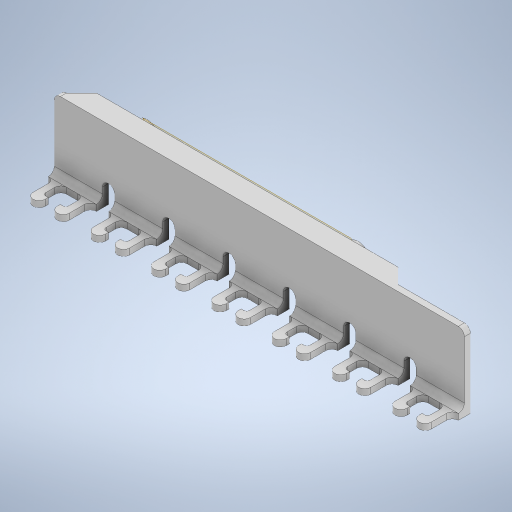
# Autodesk Inventor part: DCB2_CableClip
Saved by Autodesk Inventor 2024.3 (Build 283343000, 343)
## iProperties
Created: 2024-05-18
Part Number: DCB2_CableClip
Material: Generic
Document SubType Name: Modeling
Designer: atrus
Density: 1 g/cm^3
Appearance: Default
Author: atrus
Autodesk Inventor part; units mm, degrees
ref_plane "YZ Plane" through (0, 0, 0) normal (1, 0, 0) x (0, 1, 0)
ref_plane "XZ Plane" through (0, 0, 0) normal (0, 1, 0) x (-1, 0, 0)
ref_plane "XY Plane" through (0, 0, 0) normal (0, 0, 1) x (1, 0, 0)
ref_plane "Work Plane1" through (0, 0, 0) normal (0, 0, 1) x (1, 0, 0)
sketch "Sketch1" plane through (0, 0, 0) normal (0, 0, 1) x (1, 0, 0)
  line L0 (19.6661, -71) -> (82.3339, -71) construction
  line L1 (82.3339, -81) -> (19.6661, -81) construction
  line L2 (1, -71) -> (101, -71)
  line L3 (101, -71) -> (101, -81)
  line L4 (101, -81) -> (1, -81)
  line L5 (1, -81) -> (1, -71)
  point P0 (0, 0)
  point P1 (51, -71)
  point P2 (51, -81)
  point P3 (101, -76)
  point P4 (1, -76)
  dimension "d0" = 100
  constraints: 8 end point, 6 midpoint, 2 parallel, 1 horizontal, 1 perpendicular
  measures "d0" distance of point (101, -76) point (1, -76)
extrude "Extrusion1" add sketch "Sketch1" along normal blind 5
sketch "Sketch2" plane through (0, 0, 5) normal (0, 0, 1) x (1, 0, 0)
  line L0 (130.0002, -96) -> (-5.9998, -96)
  line L1 (-5.9998, -96) -> (-5.9998, -71)
  line L2 (-5.9998, -71) -> (130.0002, -71)
  line L3 (130.0002, -71) -> (130.0002, -96)
  line L4 (-2.4998, -51.4004) -> (-2.4998, -61.4004) projected
  line L5 (126.5002, -51.4004) -> (126.5002, -61.4004) projected
  line L6 (101, -71) -> (1, -71) projected
  point P0 (0, 0)
  point P1 (-2.4998, -56.4004)
  point P2 (130.0002, -83.5)
  point P3 (51, -71)
  dimension "d3" = 3.5
  dimension "d4" = 3.5
  dimension "d5" = 25
  constraints: 8 end point, 3 midpoint, 2 parallel, 1 horizontal, 1 perpendicular, 1 point on line
  measures "d3" distance from line of point (-2.5, -56.4) L1
  measures "d4" distance from line of point (130, -83.5) L5
  measures "d5" distance of L0.end L1.end
extrude "Extrusion2" add sketch "Sketch2" along normal blind 2
sketch "Sketch3" plane through (0, 0, 7) normal (0, 0, 1) x (1, 0, 0)
  line L0 (-2.4998, -63.9004) -> (6.5002, -63.9004)
  line L1 (17.5002, -63.9004) -> (26.5002, -63.9004)
  line L2 (37.5002, -63.9004) -> (46.5002, -63.9004)
  line L3 (57.5002, -63.9004) -> (66.5002, -63.9004)
  line L4 (77.5002, -63.9004) -> (86.5002, -63.9004)
  line L5 (97.5002, -63.9004) -> (106.5002, -63.9004)
  line L6 (117.5002, -63.9004) -> (126.5002, -63.9004)
  line L7 (2.0002, -63.9004) -> (2.0002, -96) construction
  line L8 (-5.9998, -96) -> (130.0002, -96) construction
  line L9 (22.0002, -63.9004) -> (22.0002, -96) construction
  line L10 (42.0002, -63.9004) -> (42.0002, -111) construction
  line L11 (62.0002, -63.9004) -> (62.0002, -96) construction
  line L12 (82.0002, -63.9004) -> (82.0002, -96) construction
  line L13 (102.0002, -63.9004) -> (102.0002, -96) construction
  line L14 (122.0002, -63.9004) -> (122.0002, -96) construction
  line L15 (-5.9998, -94) -> (10.0002, -94)
  line L16 (10.0002, -94) -> (10.0002, -96)
  line L17 (10.0002, -96) -> (-5.9998, -96)
  line L18 (-5.9998, -96) -> (-5.9998, -94)
  line L19 (30.0002, -94) -> (30.0002, -96)
  line L20 (14.0002, -94) -> (30.0002, -94)
  line L21 (30.0002, -96) -> (14.0002, -96)
  line L22 (14.0002, -96) -> (14.0002, -94)
  line L23 (50.0002, -94) -> (50.0002, -96)
  line L24 (34.0002, -94) -> (50.0002, -94)
  line L25 (50.0002, -96) -> (34.0002, -96)
  line L26 (34.0002, -96) -> (34.0002, -94)
  line L27 (70.0002, -94) -> (70.0002, -96)
  line L28 (54.0002, -94) -> (70.0002, -94)
  line L29 (70.0002, -96) -> (54.0002, -96)
  line L30 (54.0002, -96) -> (54.0002, -94)
  line L31 (90.0002, -94) -> (90.0002, -96)
  line L32 (74.0002, -94) -> (90.0002, -94)
  line L33 (90.0002, -96) -> (74.0002, -96)
  line L34 (74.0002, -96) -> (74.0002, -94)
  line L35 (110.0002, -94) -> (110.0002, -96)
  line L36 (94.0002, -94) -> (110.0002, -94)
  line L37 (110.0002, -96) -> (94.0002, -96)
  line L38 (94.0002, -96) -> (94.0002, -94)
  line L39 (130.0002, -94) -> (130.0002, -96)
  line L40 (114.0002, -94) -> (130.0002, -94)
  line L41 (130.0002, -96) -> (114.0002, -96)
  line L42 (114.0002, -96) -> (114.0002, -94)
  point P0 (0, 0)
  point P1 (2.0002, -94)
  point P2 (22.0002, -94)
  point P3 (22.0002, -96)
  point P4 (42.0002, -94)
  point P5 (42.0002, -96)
  point P6 (62.0002, -94)
  point P7 (62.0002, -96)
  point P8 (82.0002, -94)
  point P9 (82.0002, -96)
  point P10 (102.0002, -94)
  point P11 (122.0002, -94)
  point P12 (122.0002, -96)
extrude "Extrusion3" add sketch "Sketch3" along normal blind 2
sketch "Sketch4" plane through (-5.9998, -96, 5) normal (0, -1, 0) x (1, 0, 0)
  line L0 (0, 4) -> (16, 4) construction
  line L1 (8, 4) -> (8, 21.3357) construction
  line L2 (2, 4) -> (2, 11)
  line L3 (4, 13) -> (4, 13)
  line L4 (6, 11) -> (6, 10)
  line L5 (6, 10) -> (5.2, 10)
  line L6 (4.2, 9) -> (4.2, 6)
  arc A0 (5.2, 10) -> (4.2, 9) centre (5.2, 9) ccw
  arc A1 (6, 11) -> (4, 13) centre (4, 11) ccw
  arc A2 (4, 13) -> (2, 11) centre (4, 11) ccw
  line L7 (0, 2) -> (0, 4) projected
  line L8 (2, 4) -> (4.2, 4)
  arc A3 (4.2, 6) -> (6.2, 4) centre (6.2, 6) ccw
  line L9 (4.2, 4) -> (6.2, 4)
  line L10 (14, 4) -> (14, 11)
  line L11 (12, 13) -> (12, 13)
  line L12 (10, 11) -> (10, 10)
  line L13 (10, 10) -> (10.8, 10)
  line L14 (11.8, 9) -> (11.8, 6)
  arc A4 (11.8, 9) -> (10.8, 10) centre (10.8, 9) ccw
  arc A5 (12, 13) -> (10, 11) centre (12, 11) ccw
  arc A6 (14, 11) -> (12, 13) centre (12, 11) ccw
  line L15 (14, 4) -> (11.8, 4)
  arc A7 (9.8, 4) -> (11.8, 6) centre (9.8, 6) ccw
  line L16 (11.8, 4) -> (9.8, 4)
  line L17 (34, 4) -> (31.8, 4)
  arc A8 (26, 11) -> (24, 13) centre (24, 11) ccw
  line L18 (24, 13) -> (24, 13)
  arc A9 (24, 13) -> (22, 11) centre (24, 11) ccw
  line L19 (31.8, 4) -> (29.8, 4)
  arc A10 (29.8, 4) -> (31.8, 6) centre (29.8, 6) ccw
  line L20 (31.8, 9) -> (31.8, 6)
  arc A11 (31.8, 9) -> (30.8, 10) centre (30.8, 9) ccw
  line L21 (30, 10) -> (30.8, 10)
  line L22 (34, 4) -> (34, 11)
  line L23 (30, 11) -> (30, 10)
  line L24 (32, 13) -> (32, 13)
  arc A12 (34, 11) -> (32, 13) centre (32, 11) ccw
  arc A13 (32, 13) -> (30, 11) centre (32, 11) ccw
  line L25 (26, 11) -> (26, 10)
  line L26 (26, 10) -> (25.2, 10)
  arc A14 (25.2, 10) -> (24.2, 9) centre (25.2, 9) ccw
  line L27 (24.2, 9) -> (24.2, 6)
  line L28 (22, 4) -> (22, 11)
  line L29 (22, 4) -> (24.2, 4)
  line L30 (24.2, 4) -> (26.2, 4)
  arc A15 (24.2, 6) -> (26.2, 4) centre (26.2, 6) ccw
  line L31 (54, 4) -> (51.8, 4)
  arc A16 (46, 11) -> (44, 13) centre (44, 11) ccw
  line L32 (44, 13) -> (44, 13)
  arc A17 (44, 13) -> (42, 11) centre (44, 11) ccw
  line L33 (51.8, 4) -> (49.8, 4)
  arc A18 (49.8, 4) -> (51.8, 6) centre (49.8, 6) ccw
  line L34 (51.8, 9) -> (51.8, 6)
  arc A19 (51.8, 9) -> (50.8, 10) centre (50.8, 9) ccw
  line L35 (50, 10) -> (50.8, 10)
  line L36 (54, 4) -> (54, 11)
  line L37 (50, 11) -> (50, 10)
  line L38 (52, 13) -> (52, 13)
  arc A20 (54, 11) -> (52, 13) centre (52, 11) ccw
  arc A21 (52, 13) -> (50, 11) centre (52, 11) ccw
  line L39 (46, 11) -> (46, 10)
  line L40 (46, 10) -> (45.2, 10)
  arc A22 (45.2, 10) -> (44.2, 9) centre (45.2, 9) ccw
  line L41 (44.2, 9) -> (44.2, 6)
  line L42 (42, 4) -> (42, 11)
  line L43 (42, 4) -> (44.2, 4)
  line L44 (44.2, 4) -> (46.2, 4)
  arc A23 (44.2, 6) -> (46.2, 4) centre (46.2, 6) ccw
  line L45 (74, 4) -> (71.8, 4)
  arc A24 (66, 11) -> (64, 13) centre (64, 11) ccw
  line L46 (64, 13) -> (64, 13)
  arc A25 (64, 13) -> (62, 11) centre (64, 11) ccw
  line L47 (71.8, 4) -> (69.8, 4)
  arc A26 (69.8, 4) -> (71.8, 6) centre (69.8, 6) ccw
  line L48 (71.8, 9) -> (71.8, 6)
  arc A27 (71.8, 9) -> (70.8, 10) centre (70.8, 9) ccw
  line L49 (70, 10) -> (70.8, 10)
  line L50 (74, 4) -> (74, 11)
  line L51 (70, 11) -> (70, 10)
  line L52 (72, 13) -> (72, 13)
  arc A28 (74, 11) -> (72, 13) centre (72, 11) ccw
  arc A29 (72, 13) -> (70, 11) centre (72, 11) ccw
  line L53 (66, 11) -> (66, 10)
  line L54 (66, 10) -> (65.2, 10)
  arc A30 (65.2, 10) -> (64.2, 9) centre (65.2, 9) ccw
  line L55 (64.2, 9) -> (64.2, 6)
  line L56 (62, 4) -> (62, 11)
  line L57 (62, 4) -> (64.2, 4)
  line L58 (64.2, 4) -> (66.2, 4)
  arc A31 (64.2, 6) -> (66.2, 4) centre (66.2, 6) ccw
  line L59 (94, 4) -> (91.8, 4)
  arc A32 (86, 11) -> (84, 13) centre (84, 11) ccw
  line L60 (84, 13) -> (84, 13)
  arc A33 (84, 13) -> (82, 11) centre (84, 11) ccw
  line L61 (91.8, 4) -> (89.8, 4)
  arc A34 (89.8, 4) -> (91.8, 6) centre (89.8, 6) ccw
  line L62 (91.8, 9) -> (91.8, 6)
  arc A35 (91.8, 9) -> (90.8, 10) centre (90.8, 9) ccw
  line L63 (90, 10) -> (90.8, 10)
  line L64 (94, 4) -> (94, 11)
  line L65 (90, 11) -> (90, 10)
  line L66 (92, 13) -> (92, 13)
  arc A36 (94, 11) -> (92, 13) centre (92, 11) ccw
  arc A37 (92, 13) -> (90, 11) centre (92, 11) ccw
  line L67 (86, 11) -> (86, 10)
  line L68 (86, 10) -> (85.2, 10)
  arc A38 (85.2, 10) -> (84.2, 9) centre (85.2, 9) ccw
  line L69 (84.2, 9) -> (84.2, 6)
  line L70 (82, 4) -> (82, 11)
  line L71 (82, 4) -> (84.2, 4)
  line L72 (84.2, 4) -> (86.2, 4)
  arc A39 (84.2, 6) -> (86.2, 4) centre (86.2, 6) ccw
  line L73 (114, 4) -> (111.8, 4)
  arc A40 (106, 11) -> (104, 13) centre (104, 11) ccw
  line L74 (104, 13) -> (104, 13)
  arc A41 (104, 13) -> (102, 11) centre (104, 11) ccw
  line L75 (111.8, 4) -> (109.8, 4)
  arc A42 (109.8, 4) -> (111.8, 6) centre (109.8, 6) ccw
  line L76 (111.8, 9) -> (111.8, 6)
  arc A43 (111.8, 9) -> (110.8, 10) centre (110.8, 9) ccw
  line L77 (110, 10) -> (110.8, 10)
  line L78 (114, 4) -> (114, 11)
  line L79 (110, 11) -> (110, 10)
  line L80 (112, 13) -> (112, 13)
  arc A44 (114, 11) -> (112, 13) centre (112, 11) ccw
  arc A45 (112, 13) -> (110, 11) centre (112, 11) ccw
  line L81 (106, 11) -> (106, 10)
  line L82 (106, 10) -> (105.2, 10)
  arc A46 (105.2, 10) -> (104.2, 9) centre (105.2, 9) ccw
  line L83 (104.2, 9) -> (104.2, 6)
  line L84 (102, 4) -> (102, 11)
  line L85 (102, 4) -> (104.2, 4)
  line L86 (104.2, 4) -> (106.2, 4)
  arc A47 (104.2, 6) -> (106.2, 4) centre (106.2, 6) ccw
  line L87 (134, 4) -> (131.8, 4)
  arc A48 (126, 11) -> (124, 13) centre (124, 11) ccw
  line L88 (124, 13) -> (124, 13)
  arc A49 (124, 13) -> (122, 11) centre (124, 11) ccw
  line L89 (131.8, 4) -> (129.8, 4)
  arc A50 (129.8, 4) -> (131.8, 6) centre (129.8, 6) ccw
  line L90 (131.8, 9) -> (131.8, 6)
  arc A51 (131.8, 9) -> (130.8, 10) centre (130.8, 9) ccw
  line L91 (130, 10) -> (130.8, 10)
  line L92 (134, 4) -> (134, 11)
  line L93 (130, 11) -> (130, 10)
  line L94 (132, 13) -> (132, 13)
  arc A52 (134, 11) -> (132, 13) centre (132, 11) ccw
  arc A53 (132, 13) -> (130, 11) centre (132, 11) ccw
  line L95 (126, 11) -> (126, 10)
  line L96 (126, 10) -> (125.2, 10)
  arc A54 (125.2, 10) -> (124.2, 9) centre (125.2, 9) ccw
  line L97 (124.2, 9) -> (124.2, 6)
  line L98 (122, 4) -> (122, 11)
  line L99 (122, 4) -> (124.2, 4)
  line L100 (124.2, 4) -> (126.2, 4)
  arc A55 (124.2, 6) -> (126.2, 4) centre (126.2, 6) ccw
  point P0 (5.9998, -5)
  point P1 (4, 13)
  point P2 (5.6, 10)
  point P3 (12, 13)
  point P4 (10.4, 10)
  point P5 (24, 13)
  point P6 (28, 4)
  point P7 (30.4, 10)
  point P8 (32, 13)
  point P9 (25.6, 10)
  point P10 (44, 13)
  point P11 (48, 4)
  point P12 (50.4, 10)
  point P13 (52, 13)
  point P14 (45.6, 10)
  point P15 (64, 13)
  point P16 (68, 4)
  point P17 (70.4, 10)
  point P18 (72, 13)
  point P19 (65.6, 10)
  point P20 (84, 13)
  point P21 (88, 4)
  point P22 (90.4, 10)
  point P23 (92, 13)
  point P24 (85.6, 10)
  point P25 (104, 13)
  point P26 (108, 4)
  point P27 (110.4, 10)
  point P28 (112, 13)
  point P29 (105.6, 10)
  point P30 (124, 13)
  point P31 (128, 4)
  point P32 (130.4, 10)
  point P33 (132, 13)
  point P34 (125.6, 10)
  point P35 (4, 13)
  point P36 (132, 13)
  point P37 (124, 13)
  point P38 (112, 13)
  point P39 (104, 13)
  point P40 (92, 13)
  point P41 (84, 13)
  point P42 (72, 13)
  point P43 (64, 13)
  point P44 (52, 13)
  point P45 (44, 13)
  point P46 (32, 13)
  point P47 (24, 13)
  point P48 (12, 13)
  dimension "d19" = 1
  dimension "d20" = 2
  dimension "d21" = 4
  dimension "d22" = 9
  dimension "d23" = 6
  dimension "d24" = 2.2
  dimension "d70" = 2
  dimension "d71" = 2
  dimension "d74" = 20
  constraints: 198 end point, 112 point on circle, 56 centre point, 17 symmetric about line, 16 point on line, 8 tangent, 4 perpendicular, 3 midpoint, 2 collinear, 2 vertical, 1 concentric, 1 horizontal, 346 other
  measures "d19" radius of A0
  measures "d20" radius of A1
  measures "d21" distance from line of L2 L4.end
  measures "d22" distance from line of L0 point (4, 13)
  measures "d23" distance from line of L0 point (5.6, 10)
  measures "d24" distance between parallel lines of L2 L6
  measures "d70" distance from line of L0.start L2
  measures "d71" radius of A3
  measures "d74" distance of L16.start L17.end
extrude "Extrusion4" add sketch "Sketch4" against normal blind 2
fillet "Fillet1" radius 2 7 edges at (2.0002, -94, 7) (22.0002, -94, 7) (42.0002, -94, 7) (62.0002, -94, 7) (82.0002, -94, 7) (102.0002, -94, 7) (122.0002, -94, 7)
fillet "Fillet2" radius 2 2 edges at (-5.9998, -71, 6) (130.0002, -71, 6)
sketch "Sketch7" plane through (0, 0, 0) normal (0, 0, -1) x (-1, 0, 0)
  circle A0 centre (-16, -76) radius 4.2 construction
  circle A1 centre (-86, -76) radius 4.2 construction
  circle A2 centre (-16, -76) radius 4
  circle A3 centre (-86, -76) radius 4
  point P0 (0, 0)
  dimension "d52" = 0.2
  constraints: 2 centre point, 2 coincident, 1 equal radius
  measures "d52" radial gap between concentric circles of A0 A2
extrude "Extrusion6" add sketch "Sketch7" along normal blind 1.8
sketch "Sketch6" plane through (0, 0, -1.8) normal (0, 0, -1) x (-1, 0, 0)
  circle A0 centre (-16, -76) radius 1.8 construction
  line L0 (-1, -81) -> (-101, -81) construction
  line L1 (-1, -71) -> (-1, -81) construction
  line L2 (-101, -71) -> (-1, -71) construction
  line L3 (-101, -81) -> (-101, -71) construction
  circle A1 centre (-86, -76) radius 1.8 construction
  circle A2 centre (-16, -76) radius 2
  circle A3 centre (-86, -76) radius 2
  point P0 (0, 0)
  dimension "d51" = 4
  constraints: 2 centre point, 2 coincident, 1 equal radius
  measures "d51" diameter of A2
extrude "Extrusion7" cut sketch "Sketch6" against normal blind 7
sketch "Sketch9" plane through (0, 0, 5) normal (0, 0, -1) x (-1, 0, 0)
  line L0 (-130.0002, -96) -> (-130.0002, -73) construction
  line L1 (-130.0002, -88) -> (5.9998, -88) construction
  line L2 (5.9998, -73) -> (5.9998, -96) construction
  line L3 (-114.0002, -96) -> (-110.0002, -96)
  line L4 (-110.0002, -96) -> (-110.0002, -88)
  line L5 (-110.0002, -88) -> (-114.0002, -88)
  line L6 (-114.0002, -88) -> (-114.0002, -96)
  line L7 (-94.0002, -96) -> (-90.0002, -96)
  line L8 (-90.0002, -96) -> (-90.0002, -88)
  line L9 (-90.0002, -88) -> (-94.0002, -88)
  line L10 (-94.0002, -88) -> (-94.0002, -96)
  line L11 (-74.0002, -96) -> (-70.0002, -96)
  line L12 (-70.0002, -96) -> (-70.0002, -88)
  line L13 (-70.0002, -88) -> (-74.0002, -88)
  line L14 (-74.0002, -88) -> (-74.0002, -96)
  line L15 (-54.0002, -96) -> (-50.0002, -96)
  line L16 (-50.0002, -96) -> (-50.0002, -88)
  line L17 (-50.0002, -88) -> (-54.0002, -88)
  line L18 (-54.0002, -88) -> (-54.0002, -96)
  line L19 (-34.0002, -96) -> (-30.0002, -96)
  line L20 (-30.0002, -96) -> (-30.0002, -88)
  line L21 (-30.0002, -88) -> (-34.0002, -88)
  line L22 (-34.0002, -88) -> (-34.0002, -96)
  line L23 (-14.0002, -96) -> (-10.0002, -96)
  line L24 (-10.0002, -96) -> (-10.0002, -88)
  line L25 (-10.0002, -88) -> (-14.0002, -88)
  line L26 (-14.0002, -88) -> (-14.0002, -96)
  line L27 (5.9998, -96) -> (-130.0002, -96) projected
  point P0 (0, 0)
  dimension "d62" = 20
  dimension "d83" = 8
  constraints: 50 end point, 9 point on line, 3 horizontal, 2 parallel, 1 perpendicular, 46 other
  measures "d62" distance of L4.end L8.end
extrude "Extrusion9" cut sketch "Sketch9" against normal blind 2
fillet "Fillet4" radius 2 12 edges at (114.0002, -88, 6) (110.0002, -88, 6) (90.0002, -88, 6) (94.0002, -88, 6) (74.0002, -88, 6) (54.0002, -88, 6) (34.0002, -88, 6) (14.0002, -88, 6) (70.0002, -88, 6) (50.0002, -88, 6) (30.0002, -88, 6) (10.0002, -88, 6)
fillet "Fillet5" radius 2 14 edges at (-3.9998, -95, 9) (8.0002, -95, 9) (16.0002, -95, 9) (28.0002, -95, 9) (48.0002, -95, 9) (68.0002, -95, 9) (88.0002, -95, 9) (108.0002, -95, 9) (128.0002, -95, 9) (116.0002, -95, 9) (96.0002, -95, 9) (76.0002, -95, 9) (56.0002, -95, 9) (36.0002, -95, 9)
chamfer "Chamfer3" distance 5 angle 45 3 edges at (101, -76, 5) (51, -81, 5) (1, -76, 5)
body "Solid1"
